Autodesk Fusion 360 part; units mm, degrees
(part 2 of 2)
sketch "Sketch2" plane through (3, 0, 0) normal (1, 0, 0) x (0, 1, 0)
  spline S0 degree 5 poles (35, 49.4017) (34.5671, 49.7896) (33.6897, 50.5546) (32.3391, 51.6696) (30.4956, 53.1165) (28.2652, 54.9855) (26.2784, 57.0434) (24.6758, 59.3564) (23.5164, 61.869) (22.719, 64.3332) (22.0218, 66.2667) (21.1315, 67.1936) (19.8358, 66.8284) (18.1658, 65.3445) (16.4091, 63.3865) (14.9295, 61.7511) (14.0473, 61.1728) (13.8699, 62.0243) (14.2266, 64.192) (14.8056, 67.2875) (15.2521, 70.7939) (15.2712, 74.2227) (14.7555, 77.3008) (13.7866, 79.9925) (12.5455, 82.3999) (11.2515, 84.7018) (10.0863, 87.0739) (9.133, 89.625) (8.2877, 92.3076) (7.2959, 94.944) (5.9556, 97.101) (4.3974, 98.4448) (2.9354, 99.1792) (1.9018, 99.5342) (1.5, 99.6524) knots 0 0 0 0 0 0 0.033333 0.066667 0.1 0.133333 0.166667 0.2 0.233333 0.266667 0.3 0.333333 0.366667 0.4 0.433333 0.466667 0.5 0.533333 0.566667 0.6 0.633333 0.666667 0.7 0.733333 0.766667 0.8 0.833333 0.866667 0.9 0.933333 0.966667 0.986276 0.986276 0.986276 0.986276 0.986276 0.986276
  line L0 (1.5, 99.6524) -> (1.5, 49.4017)
  line L1 (1.5, 49.4017) -> (-1.5, 49.4017)
  line L2 (-1.5, 49.4017) -> (-1.5, 99.6524)
  spline S1 degree 5 poles (-1.5, 99.6524) (-1.9018, 99.5342) (-2.9354, 99.1792) (-4.3974, 98.4448) (-5.9556, 97.101) (-7.2959, 94.944) (-8.2877, 92.3076) (-9.133, 89.625) (-10.0863, 87.0739) (-11.2515, 84.7018) (-12.5455, 82.3999) (-13.7866, 79.9925) (-14.7555, 77.3008) (-15.2712, 74.2227) (-15.2521, 70.7939) (-14.8056, 67.2875) (-14.2266, 64.192) (-13.8699, 62.0243) (-14.0473, 61.1728) (-14.9295, 61.7511) (-16.4091, 63.3865) (-18.1658, 65.3445) (-19.8358, 66.8284) (-21.1315, 67.1936) (-22.0218, 66.2667) (-22.719, 64.3332) (-23.5164, 61.869) (-24.6758, 59.3564) (-26.2784, 57.0434) (-28.2652, 54.9855) (-30.4956, 53.1165) (-32.3391, 51.6696) (-33.6897, 50.5546) (-34.5671, 49.7896) (-35, 49.4017) knots -0.986276 -0.986276 -0.986276 -0.986276 -0.986276 -0.986276 -0.966667 -0.933333 -0.9 -0.866667 -0.833333 -0.8 -0.766667 -0.733333 -0.7 -0.666667 -0.633333 -0.6 -0.566667 -0.533333 -0.5 -0.466667 -0.433333 -0.4 -0.366667 -0.333333 -0.3 -0.266667 -0.233333 -0.2 -0.166667 -0.133333 -0.1 -0.066667 -0.033333 0 0 0 0 0 0
  line L3 (-35, 49.4017) -> (-35, 0.4017)
  line L4 (-35, 0.4017) -> (35, 0.4017)
  line L5 (35, 0.4017) -> (35, 49.4017)
equation "d10 = ( 70 / 2 ) * 1 mm"
equation "d12 = ( 3 / 2 ) * 1 mm"

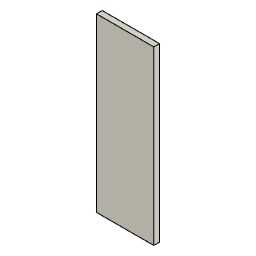
design "_water_level_sensor"
Autodesk Fusion 360 part; units mm, degrees
sketch "Sketch1" plane through (0, 0, 0) normal (0, 1, 0) x (1, 0, 0)
  line L0 (0, 0) -> (20, 0)
  line L1 (20, 0) -> (20, -60)
  line L2 (20, -60) -> (0, -60)
  line L3 (0, -60) -> (0, 0)
  dimension "d1" = 20
  dimension "d2" = 60
  constraint horizontal L0
  constraint vertical L1
  constraint horizontal L2
  constraint vertical L3
  constraint coincident L0.start L3.end
  measures "d1" distance of L0.start L0.end
  measures "d2" distance of L0.start L2.end
extrude "Extrude1" add sketch "Sketch1" along normal blind 2

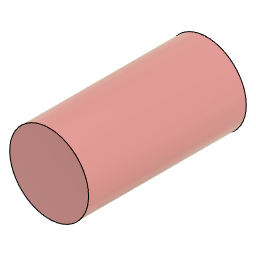
design "_per_pump"
Autodesk Fusion 360 part; units mm, degrees
sketch "Sketch1" plane through (0, 0, 0) normal (0, 1, 0) x (1, 0, 0)
  circle A0 centre (0, 0) radius 15
  dimension "d1" = 30
  constraint coincident A0.centre origin
  measures "d1" diameter of A0
extrude "Extrude1" add sketch "Sketch1" along normal blind 60

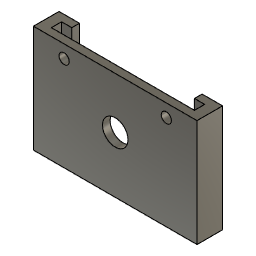
design "SolarPanelHolder"
Autodesk Fusion 360 part; units mm, degrees
sketch "Sketch1" plane through (0, 0, 0) normal (0, 1, 0) x (1, 0, 0)
  line L0 (0, -52.4738) -> (0, 26.7637) construction
  line L1 (-32, 0) -> (-32, -42)
  line L2 (0, 0) -> (-32, 0)
  line L3 (-32, -42) -> (0, -42)
  line L4 (32, 0) -> (32, -42)
  line L5 (32, -42) -> (0, -42)
  line L6 (0, 0) -> (32, 0)
  dimension "d1" = 32
  dimension "d2" = 42
  constraint vertical L0
  constraint vertical L1
  constraint coincident L2.start L6.start
  constraint perpendicular L1 L2
  constraint coincident L0 L3.end
  constraint perpendicular L0 L3
  constraint symmetric L0 L1.start L4.start
  constraint symmetric L0 L1.end L4.end
  constraint symmetric L0 L2.start L6.start
  constraint symmetric L0 L3.end L5.end
  measures "d1" distance of L0 L1
  measures "d2" distance of L1.start L1.end
extrude "Extrude1" add sketch "Sketch1" along normal blind 10
sketch "Sketch2" plane through (0, 0, 42) normal (0, 0, 1) x (-1, 0, 0)
  line L0 (32, 0) -> (-32, 0)
  line L1 (-32, 0) -> (-32, -10)
  line L2 (-32, -10) -> (32, -10)
  line L3 (32, -10) -> (32, 0)
  line L4 (-36, -5) -> (37, -5) construction
  line L5 (32, -3) -> (-32, -3)
  line L6 (28, 0) -> (28, -10)
  line L7 (0, -15) -> (0, 7) construction
  line L8 (32, -7) -> (-32, -7)
  line L9 (-28, 0) -> (-28, -10)
  dimension "d5" = 5
  dimension "d6" = 2
  dimension "d7" = 4
  dimension "d21" = 28
  constraint perpendicular L1 L4
  constraint coincident L3 L5.start
  constraint coincident L1 L5.end
  constraint perpendicular L1 L5
  constraint coincident L0 L6.start
  constraint coincident L2 L6.end
  constraint perpendicular L2 L6
  constraint perpendicular L2 L7
  constraint symmetric L4 L5.start L8.start
  constraint symmetric L4 L5.end L8.end
  constraint symmetric L6.start L7 L9.start
  constraint symmetric L6.end L7 L9.end
  measures "d5" distance of L0 L4
  measures "d6" distance of L4 L5
  measures "d7" distance of L3 L6
  measures "d21" distance of L6 L7
extrude "Extrude2" cut sketch "Sketch2" against normal blind 40 contours L5 L6 L8 L9
sketch "Sketch3" plane through (0, 10, 0) normal (0, 1, 0) x (-1, 0, 0)
  line L0 (32, 0) -> (32, 42)
  line L1 (32, 42) -> (-32, 42)
  line L2 (-32, 42) -> (-32, 0)
  line L3 (-32, 0) -> (32, 0)
  line L4 (0, 44) -> (0, 0) construction
  line L5 (24, 42) -> (24, 0)
  line L6 (-24, 42) -> (-24, 0)
  line L7 (-32, 2) -> (32, 2)
  dimension "d10" = 24
  dimension "d11" = 40
  constraint coincident L4.end origin
  constraint perpendicular L3 L4
  constraint perpendicular L3 L5
  constraint coincident L3 L5.end
  constraint coincident L1 L5.start
  constraint symmetric L4 L5.start L6.start
  constraint symmetric L4 L5.end L6.end
  constraint coincident L2 L7.start
  constraint coincident L0 L7.end
  constraint perpendicular L0 L7
  measures "d10" distance of L4 L5
  measures "d11" distance of L1 L7
extrude "Extrude3" cut sketch "Sketch3" against normal blind 3 contours L1 L5 L6 L7
sketch "Sketch4" plane through (0, 0, 0) normal (0, 1, 0) x (1, 0, 0)
  line L0 (0, -44) -> (0, 0) construction
  line L1 (-36, -37) -> (36, -37) construction
  line L2 (-32, -42) -> (32, -42)
  line L3 (-20, -44) -> (-20, -33) construction
  circle A0 centre (-20, -37) radius 2
  circle A1 centre (20, -37) radius 2
  line L4 (-40, -22) -> (39, -22) construction
  line L5 (-28, -42, 3) -> (28, -42, 3)
  line L6 (28, -42, 3) -> (28, -2, 3)
  line L7 (28, -2, 3) -> (-28, -2, 3)
  line L8 (-28, -2, 3) -> (-28, -42, 3)
  circle A2 centre (0, -22) radius 5
  dimension "d14" = 5
  dimension "d15" = 20
  dimension "d16" = 4
  dimension "d20" = 10
  dimension "d22" = 15
  constraint coincident L0.end origin
  constraint vertical L0
  constraint horizontal L1
  constraint perpendicular L1 L3
  constraint coincident L3 A0.centre
  constraint coincident L1 A0.centre
  constraint symmetric L0 A0 A1
  constraint horizontal L4
  constraint midpoint L0 A2.centre
  measures "d14" distance of L1 L2
  measures "d15" distance of L0 L3
  measures "d16" diameter of A0
  measures "d20" diameter of A2
  measures "d22" distance of L1 L4
extrude "Extrude4" cut sketch "Sketch4" along normal blind 3
equation "d1 = ( ( 54 + 10 ) / 2 ) * 1 mm"
equation "d2 = 32 mm + 10 mm"
equation "d10 = ( 48 / 2 ) * 1 mm"

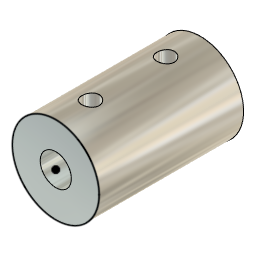
design "MotorShaft_Screw_Fixer"
Autodesk Fusion 360 part; units mm, degrees
sketch "Sketch1" plane through (0, 0, 0) normal (0, 1, 0) x (1, 0, 0)
  circle A0 centre (0, 0) radius 7.5
  dimension "d1" = 15
  constraint coincident A0.centre origin
  measures "d1" diameter of A0
extrude "Extrude7" add sketch "Sketch1" along normal blind 25
sketch "Sketch6" plane through (0, 0, 0) normal (0, 1, 0) x (1, 0, 0)
  circle A0 centre (0, 0) radius 2.7
  dimension "d29" = 5.4
  constraint coincident A0.centre origin
  measures "d29" diameter of A0
extrude "Extrude8" cut sketch "Sketch6" along normal blind 10
ref_plane "WorkPlane3" through (0, 4.7948, 7.5) normal (0, 0, 1) x (-1, 0, 0)
sketch "Sketch7" plane through (0, 0, 7.5) normal (0, 0, 1) x (1, 0, 0)
  line L0 (0, 0) -> (0, 6) construction
  circle A0 centre (0, 6) radius 1.5
  dimension "d33" = 6
  dimension "d34" = 3
  constraint coincident L0.start origin
  constraint vertical L0
  constraint coincident L0.end A0.centre
  measures "d33" distance of L0.start L0.end
  measures "d34" diameter of A0
extrude "Extrude9" cut sketch "Sketch7" against normal blind 6
sketch "Sketch8" plane through (0, 25, 0) normal (0, 1, 0) x (-1, 0, 0)
  circle A0 centre (0, 0) radius 7.5
  circle A1 centre (0, 0) radius 2.15
  dimension "d37" = 4.3
  constraint coincident A0.centre A1.centre
  measures "d37" diameter of A1
extrude "Extrude10" cut sketch "Sketch8" against normal blind 10 contours A1
ref_plane "WorkPlane4" through (0, 19.902, 7.5) normal (0, 0, 1) x (-1, 0, 0)
sketch "Sketch9" plane through (0, 0, 7.5) normal (0, 0, 1) x (1, 0, 0)
  line L0 (0, 25) -> (0, 19) construction
  circle A0 centre (0, 19) radius 1.5
  dimension "d41" = 6
  dimension "d42" = 3
  constraint vertical L0
  constraint coincident L0.end A0.centre
  measures "d41" distance of L0.start L0.end
  measures "d42" diameter of A0
extrude "Extrude11" cut sketch "Sketch9" against normal blind 7

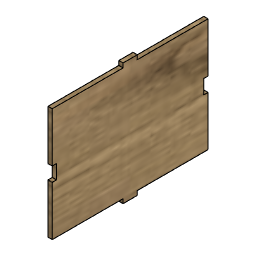
design "ShortWall_"
Autodesk Fusion 360 part; units mm, degrees
sketch "Sketch2" plane through (0, 0, 0) normal (1, 0, 0) x (0, 1, 0)
  line L0 (0, 80) -> (55, 80)
  line L1 (55, 40) -> (0, 40)
  line L2 (0, 80) -> (-55, 80)
  line L3 (5, 80) -> (5, 83)
  line L4 (-5, 80) -> (-5, 83)
  line L5 (5, 83) -> (0, 83)
  line L6 (0, 83) -> (0, 80)
  line L7 (-5, 83) -> (0, 83)
  line L8 (55, 40) -> (0, 40)
  line L9 (52, 35) -> (55, 35)
  line L10 (52, 40) -> (52, 45)
  line L11 (55, 0) -> (55, 40)
  line L12 (52, 40) -> (52, 35)
  line L13 (-5, -3) -> (0, -3)
  line L14 (-55, 40) -> (-52, 40)
  line L15 (-55, 40) -> (-52, 40)
  line L16 (-5, 0) -> (-5, -3)
  line L17 (-55, 45) -> (-55, 40)
  line L18 (-52, 40) -> (-52, 45)
  line L19 (5, -3) -> (0, -3)
  line L20 (-52, 45) -> (-55, 45)
  line L21 (0, 0) -> (55, 0)
  line L22 (0, 80) -> (-5, 80)
  line L23 (0, 40) -> (0, 80)
  line L24 (-55, 40) -> (0, 40)
  line L25 (0, 40) -> (0, 0)
  line L26 (0, 80) -> (5, 80)
  line L27 (0, 83) -> (0, 80)
  line L28 (55, 80) -> (55, 40)
  line L29 (55, 40) -> (52, 40)
  line L30 (55, 40) -> (52, 40)
  line L31 (55, 35) -> (55, 40)
  line L32 (0, 40) -> (0, 80)
  line L33 (55, 45) -> (55, 40)
  line L34 (-55, 40) -> (0, 40)
  line L35 (52, 45) -> (55, 45)
  line L36 (0, 40) -> (0, 0)
  line L37 (5, 0) -> (5, -3)
  line L38 (0, -3) -> (0, 0)
  line L39 (0, 0) -> (-55, 0)
  line L40 (-55, 0) -> (-55, 40)
  line L41 (0, 0) -> (5, 0)
  line L42 (-55, 80) -> (-55, 40)
  line L43 (0, -3) -> (0, 0)
  line L44 (-52, 35) -> (-55, 35)
  line L45 (-52, 40) -> (-52, 35)
  line L46 (-55, 35) -> (-55, 40)
  line L47 (0, 0) -> (-5, 0)
  point P0 (0, 80)
  point P1 (0, 80)
  dimension "d1" = 55
  dimension "d2" = 40
  dimension "d3" = 3
  dimension "d4" = 5
  dimension "d5" = 5
  dimension "d6" = 3
  constraint horizontal L21
  constraint vertical L11
  constraint horizontal L1
  constraint vertical L25
  constraint coincident L21.start L25.end
  constraint horizontal L29
  constraint vertical L12
  constraint horizontal L9
  constraint vertical L31
  constraint horizontal L41
  constraint vertical L37
  constraint horizontal L19
  constraint vertical L38
  constraint symmetric L21.start L36.end L25
  constraint symmetric L11.start L39.end L25
  constraint symmetric L1.start L14.start L25
  constraint symmetric L1.end L8.end L25
  constraint symmetric L14.end L10.start L25
  constraint symmetric L44.start L9.start L25
  constraint symmetric L44.end L9.end L25
  constraint symmetric L16.start L37.start L25
  constraint symmetric L13.start L19.start L25
  constraint symmetric L13.end L19.end L25
  constraint symmetric P1 L21.start L1
  constraint symmetric L0.end L11.start L1
  constraint symmetric L8.start L11.end L1
  constraint symmetric L8.end L23.start L1
  constraint symmetric L10.start L12.start L1
  constraint symmetric L10.end L9.start L1
  constraint symmetric L33.start L9.end L1
  constraint symmetric L3.start L37.start L1
  constraint symmetric L3.end L19.start L1
  constraint symmetric L5.end L13.end L1
  constraint symmetric L4.end L13.start L1
  constraint symmetric L2.end L39.end L1
  constraint symmetric L14.end L15.end L1
  constraint symmetric L14.start L15.start L1
  constraint symmetric L17.start L44.end L1
  constraint symmetric L18.end L44.start L1
  constraint symmetric L4.start L16.start L1
  constraint symmetric P0 L21.start L1
  measures "d1" distance of L21.start L11.start
  measures "d2" distance of L21.start L1.end
  measures "d3" distance of L1.start L10.start
  measures "d4" distance of L1.start L9.end
  measures "d5" distance of L21.start L37.start
  measures "d6" distance of L21.start L13.end
extrude "Extrude1" add sketch "Sketch2" along normal blind 3 contours L0 L3 L5 L6 L26 L27 | L2 L18 L20 L22 L23 L24 L32 L34 L42 | L2 L4 L6 L7 L22 L27 | L0 L1 L8 L10 L23 L26 L28 L32 L35 | L24 L25 L34 L36 L39 L40 L44 L45 L47 | L1 L8 L9 L11 L12 L21 L25 L36 L41 | L19 L21 L37 L38 L41 L43 | L13 L16 L38 L39 L43 L47
ref_plane "WorkPlane1" through (3, 0, 40) normal (1, 0, 0) x (0, 0, -1)
sketch "Sketch3" plane through (3, 0, 0) normal (1, 0, 0) x (0, 1, 0)

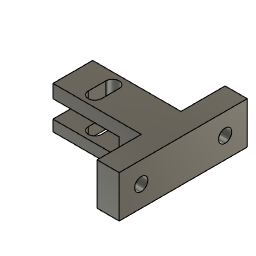
design "IR_Sensor_Holder"
Autodesk Fusion 360 part; units mm, degrees
sketch "Sketch1" plane through (0, 0, 0) normal (0, 0, 1) x (1, 0, 0)
  line L0 (0, 0) -> (0, 9)
  line L1 (0, 0) -> (25, 0)
  line L2 (25, 0) -> (25, 9)
  line L3 (0, 9) -> (25, 9)
  line L4 (7, 12) -> (7, -6) construction
  line L5 (4.5, 6.5) -> (11.5, 6.5) construction
  line L6 (4.5, 2.5) -> (12.5, 2.5) construction
  circle A0 centre (7, 6.5) radius 1.5
  circle A1 centre (7, 2.5) radius 1.5
  line L7 (5.5, 6.5) -> (5.5, 2.5)
  line L8 (8.5, 6.5) -> (8.5, 2.5)
  dimension "d2" = 9
  dimension "d3" = 25
  dimension "d4" = 9
  dimension "d5" = 7
  dimension "d8" = 2.5
  dimension "d9" = 2.5
  dimension "d10" = 3
  dimension "d12" = 3
  constraint coincident L0.start L1.start
  constraint vertical L0
  constraint perpendicular L0 L1
  constraint perpendicular L1 L2
  constraint vertical L4
  constraint horizontal L5
  constraint horizontal L6
  constraint coincident L4 A0.centre
  constraint coincident L5 A0.centre
  constraint coincident L6 A1.centre
  constraint coincident L4 A1.centre
  constraint coincident A0 L7.start
  constraint coincident L5 L7.start
  constraint coincident A1 L7.end
  constraint coincident L6 L7.end
  constraint coincident A0 L8.start
  constraint coincident L5 L8.start
  constraint midpoint L6 L8.end
  measures "d2" distance of L0.start L0.end
  measures "d3" distance of L0.start L1.end
  measures "d4" distance of L1.end L2.end
  measures "d5" distance of L0 L4
  measures "d8" distance of L3 L5
  measures "d9" distance of L1 L6
  measures "d10" diameter of A0
  measures "d12" diameter of A1
extrude "Extrude1" add sketch "Sketch1" against normal blind 9.5
sketch "Sketch2" plane through (0, 9, 0) normal (0, 1, 0) x (-1, 0, 0)
  line L0 (0, 0) -> (-25, 0)
  line L1 (-25, 0) -> (-25, -9.5)
  line L2 (-25, -9.5) -> (0, -9.5)
  line L3 (0, -9.5) -> (0, 0)
  line L4 (2, -5) -> (-23, -5) construction
  line L5 (-15, -9.5) -> (-15, 0)
  line L6 (0, -3) -> (-15, -3)
  line L7 (0, -7) -> (-15, -7)
  line L8 (0, -7) -> (0, -3)
  dimension "d15" = 5
  dimension "d16" = 15
  dimension "d17" = 2
  constraint horizontal L4
  constraint coincident L2 L5.start
  constraint coincident L0 L5.end
  constraint perpendicular L0 L5
  constraint coincident L3 L6.start
  constraint coincident L5 L6.end
  constraint perpendicular L5 L6
  constraint symmetric L4 L6.start L7.start
  constraint symmetric L4 L6.end L7.end
  measures "d15" distance of L0 L4
  measures "d16" distance of L3 L5
  measures "d17" distance of L4 L6
extrude "Extrude2" cut sketch "Sketch2" against normal blind 9 contours L3 L5 L6 L7 L8
sketch "Sketch3" plane through (0, 0, -9.5) normal (0, 0, -1) x (1, 0, 0)
  line L0 (5.5, -6.5) -> (5.5, -2.5)
  arc A0 (8.5, -2.5) -> (5.5, -2.5) centre (7, -2.5) ccw
  line L1 (8.5, -2.5) -> (8.5, -6.5)
  arc A1 (5.5, -6.5) -> (8.5, -6.5) centre (7, -6.5) ccw
  line L2 (25, 0) -> (0, 0)
  line L3 (0, 0) -> (0, -9)
  line L4 (0, -9) -> (25, -9)
  line L5 (25, -9) -> (25, 0)
sketch "Sketch4" plane through (25, 0, 0) normal (1, 0, 0) x (0, 1, 0)
  line L0 (9, 0) -> (0, 0)
  line L1 (0, 0) -> (0, -9.5)
  line L2 (0, -9.5) -> (9, -9.5)
  line L3 (9, -9.5) -> (9, 0)
  line L4 (9, 0) -> (19, 0)
  line L5 (19, 0) -> (19, -9.5)
  line L6 (19, -9.5) -> (9, -9.5)
  line L7 (9, -9.5) -> (9, 0)
  line L8 (19, 0) -> (9, -9.5) construction
  line L9 (9, 0) -> (19, -9.5) construction
  circle A0 centre (14, -4.75) radius 1.5
  line L10 (4.5, 2) -> (4.5, -12.7462) construction
  line L11 (0, 0) -> (-10, 0)
  line L12 (0, -9.5) -> (0, 0)
  line L13 (-10, -9.5) -> (0, -9.5)
  line L14 (-10, 0) -> (-10, -9.5)
  circle A1 centre (-5, -4.75) radius 1.5
  dimension "d20" = 10
  dimension "d21" = 9.5
  dimension "d22" = 3
  dimension "d23" = 4.5
  constraint horizontal L4
  constraint vertical L5
  constraint horizontal L6
  constraint vertical L7
  constraint coincident L0.start L3.end
  constraint coincident L2.end L3.start
  constraint midpoint L9 A0.centre
  constraint vertical L10
  constraint symmetric L0.start L10 L0.end
  constraint symmetric L4.end L10 L11.end
  constraint symmetric L5.end L10 L13.start
  constraint symmetric L2.end L10 L1.end
  constraint symmetric A0 L10 A1
  measures "d20" distance of L0.start L4.end
  measures "d21" distance of L4.end L5.end
  measures "d22" diameter of A0
  measures "d23" distance of L1 L10
extrude "Extrude3" add sketch "Sketch4" against normal blind 5 contours L3 L4 L5 L6 L7 | L1 L11 L12 L13 L14

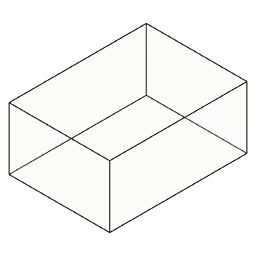
design "_WaterTank"
Autodesk Fusion 360 part; units mm, degrees
sketch "Sketch1" plane through (0, 0, 0) normal (0, 0, 1) x (1, 0, 0)
  line L0 (0, 0) -> (110, 0)
  line L1 (110, 0) -> (110, 150)
  line L2 (110, 150) -> (0, 150)
  line L3 (0, 150) -> (0, 0)
  dimension "d1" = 150
  dimension "d2" = 110
  constraint horizontal L0
  constraint vertical L1
  constraint horizontal L2
  constraint vertical L3
  constraint coincident L0.start L3.end
  measures "d1" distance of L0.start L2.end
  measures "d2" distance of L0.start L0.end
extrude "Extrude1" add sketch "Sketch1" along normal blind 68

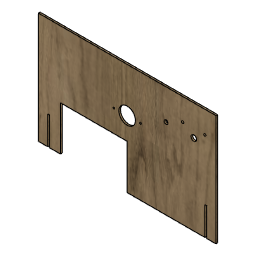
design "Base_Wall"
Autodesk Fusion 360 part; units mm, degrees
sketch "Sketch3" plane through (0, 0, 0) normal (0, 1, 0) x (1, 0, 0)
  line L0 (0, 0) -> (0, -200) construction
  line L1 (0, -200) -> (-160, -200)
  line L2 (-160, -200) -> (-160, 0)
  line L3 (-160, 0) -> (0, 0)
  line L4 (-140, -27.5484) -> (-140, 15) construction
  line L5 (-140, 0) -> (-140, -51)
  line L6 (-140, -51) -> (-143, -51)
  line L7 (-143, -51) -> (-143, 0)
  line L8 (160, -200) -> (160, 0)
  line L9 (143, -51) -> (143, 0)
  line L10 (140, 0) -> (140, -51)
  line L11 (160, 0) -> (0, 0)
  line L12 (0, -200) -> (160, -200)
  line L13 (140, -51) -> (143, -51)
  line L14 (150, -200) -> (150, -125) construction
  line L15 (131.5, -205) -> (131.5, -122.2799) construction
  line L16 (58.1813, -150) -> (105, -150) construction
  line L17 (60, -162.5) -> (118, -162.5) construction
  line L18 (-37.7512, -120) -> (47.9095, -120) construction
  circle A0 centre (0, -120) radius 15
  line L19 (-24, -155) -> (-24, -112) construction
  circle A1 centre (-24, -120) radius 1.5
  circle A2 centre (24, -120) radius 1.5
  dimension "d15" = 200
  dimension "d16" = 160
  dimension "d17" = 140
  dimension "d18" = 51
  dimension "d19" = 3
  dimension "d22" = 10
  dimension "d23" = 18.5
  dimension "d24" = 50
  dimension "d28" = 12.5
  dimension "d31" = 120
  dimension "d33" = 30
  dimension "d34" = 24
  dimension "d36" = 3
  constraint coincident L0.start L3.end
  constraint vertical L0
  constraint perpendicular L0 L1
  constraint perpendicular L1 L2
  constraint perpendicular L0 L3
  constraint perpendicular L3 L4
  constraint coincident L3 L5.start
  constraint coincident L4 L5.start
  constraint perpendicular L3 L5
  constraint perpendicular L4 L6
  constraint coincident L3 L7.end
  constraint perpendicular L3 L7
  constraint symmetric L1.start L0 L12.start
  constraint symmetric L0 L1.end L8.start
  constraint symmetric L0 L2.end L8.end
  constraint symmetric L0 L3.end L11.end
  constraint symmetric L0 L5.start L10.start
  constraint symmetric L0 L5.end L10.end
  constraint symmetric L0 L6.end L9.start
  constraint symmetric L0 L7.end L9.end
  constraint coincident L12 L14.start
  constraint perpendicular L12 L14
  constraint perpendicular L12 L15
  constraint horizontal L16
  constraint perpendicular L8 L17
  constraint perpendicular L0 L18
  constraint coincident L18 A0.centre
  constraint coincident L0 A0.centre
  constraint perpendicular L18 L19
  constraint coincident L18 A1.centre
  constraint coincident L19 A1.centre
  constraint symmetric L0 A1 A2
  measures "d15" distance of L0.start L0.end
  measures "d16" distance of L0.end L1.end
  measures "d17" distance of L0 L4
  measures "d18" distance of L5.start L5.end
  measures "d19" distance of L5.end L6.end
  measures "d22" distance of L8 L14
  measures "d23" distance of L14 L15
  measures "d24" distance of L12 L16
  measures "d28" distance of L16 L17
  measures "d31" distance of L3 L18
  measures "d33" diameter of A0
  measures "d34" distance of L0 L19
  measures "d36" diameter of A1
extrude "Extrude3" add sketch "Sketch3" along normal blind 3 contours L1 L2 L3 L5 L6 L7 L8 L9 L10 L11 L12 L13
sketch "Sketch4" plane through (0, 0, 0) normal (0, -1, 0) x (1, 0, 0)
  circle A0 centre (-24, 120) radius 1.5
  circle A1 centre (24, 120) radius 1.5
  circle A2 centre (0, 120) radius 15
  line L0 (-140, 0) -> (140, 0)
  line L1 (140, 0) -> (140, 51)
  line L2 (140, 51) -> (143, 51)
  line L3 (143, 51) -> (143, 0)
  line L4 (143, 0) -> (160, 0)
  line L5 (160, 0) -> (160, 200)
  line L6 (160, 200) -> (-160, 200)
  line L7 (-160, 200) -> (-160, 0)
  line L8 (-160, 0) -> (-143, 0)
  line L9 (-143, 0) -> (-143, 51)
  line L10 (-143, 51) -> (-140, 51)
  line L11 (-140, 51) -> (-140, 0)
  line L12 (0, 170) -> (0, -33.7558) construction
  line L13 (-60, 120) -> (-60, -60) construction
  line L14 (-120, 80) -> (-120, 0)
  line L15 (0, 80) -> (0, 0)
  line L16 (-120, 80) -> (0, 80)
  dimension "d39" = 60
  dimension "d40" = 80
  dimension "d57" = 60
  constraint vertical L12
  constraint parallel L12 L13
  constraint perpendicular L0 L14
  constraint coincident L0 L14.end
  constraint symmetric L13 L14.start L15.start
  constraint symmetric L13 L14.end L15.end
  measures "d39" distance of L13 L14
  measures "d40" distance of L14.start L14.end
  measures "d57" distance of L12 L13
extrude "Extrude4" cut sketch "Sketch4" against normal blind 3 contours L0 L14 L15 L16
sketch "Sketch5" plane through (0, 0, 0) normal (0, 1, 0) x (1, 0, 0)
  line L0 (120, -207.9791) -> (120, -95) construction
  line L1 (160, -200) -> (160, 0)
  line L2 (175, -160) -> (75, -160) construction
  line L3 (160, -200) -> (-160, -200) construction
  line L4 (77.3265, -145) -> (160, -145) construction
  circle A0 centre (120, -145) radius 5
  line L5 (140, -179) -> (140, -139) construction
  circle A1 centre (140, -160) radius 2
  circle A2 centre (100, -160) radius 2
  dimension "d43" = 40
  dimension "d44" = 40
  dimension "d45" = 15
  dimension "d46" = 10
  dimension "d47" = 20
  dimension "d48" = 4
  constraint vertical L0
  constraint perpendicular L1 L2
  constraint parallel L2 L4
  constraint coincident L4 A0.centre
  constraint coincident L0 A0.centre
  constraint perpendicular L4 L5
  constraint coincident L2 A1.centre
  constraint coincident L5 A1.centre
  constraint symmetric L0 A1 A2
  measures "d43" distance of L0 L1
  measures "d44" distance of L2 L3
  measures "d45" distance of L2 L4
  measures "d46" diameter of A0
  measures "d47" distance of L0 L5
  measures "d48" diameter of A1
extrude "Extrude5" cut sketch "Sketch5" along normal blind 3
sketch "Sketch6" plane through (0, 0, 0) normal (0, 1, 0) x (1, 0, 0)
  line L0 (70, -200) -> (70, -105.2001) construction
  line L1 (160, -200) -> (160, 0) construction
  line L2 (60, -145) -> (172.965, -145) construction
  line L3 (160, -200) -> (-160, -200) construction
  circle A0 centre (70, -145) radius 3.5
  dimension "d51" = 90
  dimension "d52" = 55
  dimension "d53" = 7
  constraint vertical L0
  constraint perpendicular L1 L2
  constraint coincident L2 A0.centre
  constraint coincident L0 A0.centre
  measures "d51" distance of L0 L1
  measures "d52" distance of L2 L3
  measures "d53" diameter of A0
extrude "Extrude6" cut sketch "Sketch6" along normal blind 3
ref_plane "WorkPlane1" through (0, 0, 0) normal (0, 1, 0) x (0, 0, 1)
sketch "Sketch7" plane through (0, 0, 0) normal (0, 1, 0) x (1, 0, 0)
  circle A0 centre (70, -145) radius 3.5
  circle A1 centre (120, -145) radius 5
  circle A2 centre (100, -160) radius 2
  circle A3 centre (140, -160) radius 2
  line L0 (0, -80) -> (0, 0)
  line L1 (0, 0) -> (140, 0)
  line L2 (140, 0) -> (140, -51)
  line L3 (140, -51) -> (143, -51)
  line L4 (143, -51) -> (143, 0)
  line L5 (143, 0) -> (160, 0)
  line L6 (160, 0) -> (160, -200)
  line L7 (160, -200) -> (-160, -200)
  line L8 (-160, -200) -> (-160, 0)
  line L9 (-160, 0) -> (-143, 0)
  line L10 (-143, 0) -> (-143, -51)
  line L11 (-143, -51) -> (-140, -51)
  line L12 (-140, -51) -> (-140, 0)
  line L13 (-140, 0) -> (-120, 0)
  line L14 (-120, 0) -> (-120, -80)
  line L15 (-120, -80) -> (0, -80)
  circle A4 centre (0, -120) radius 15
  circle A5 centre (24, -120) radius 1.5
  circle A6 centre (-24, -120) radius 1.5
equation "foot_thickness = 10 mm"
equation "d23 = ( 37 / 2 ) * 1 mm"
